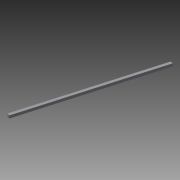
# Autodesk Inventor part: Stand
Saved by Autodesk Inventor 2017 (Build 210142000, 142)
## iProperties
Created: 2018-10-12
Part Number: Stand
Material: Wood (Birch)
Document SubType Name: Modeling
Designer: ari
Density: 0.55 g/cm^3
Appearance: Birch - Natural Polished
Author: ari
Autodesk Inventor part; units mm, degrees
ref_plane "XZ Plane" through (0, 0, 0) normal (0, 1, 0) x (-1, 0, 0)
ref_plane "XY Plane" through (0, 0, 0) normal (0, 0, 1) x (1, 0, 0)
sketch "Sketch1" plane through (0, 0, 0) normal (0, 0, 1) x (1, 0, 0)
  line L0 (-102.7252, -80.4997) -> (-34.2492, 156.7326)
  line L1 (-34.2492, 156.7326) -> (-39.0531, 158.1192)
  line L2 (-39.0531, 158.1192) -> (-107.529, -79.1131)
  line L3 (-107.529, -79.1131) -> (-102.7252, -80.4997)
  line L4 (-66.029, -80.4997) -> (-399.029, -80.4997) construction
  line L5 (-41.9395, 115.6973) -> (-41.9395, 350.8973) construction
  line L6 (-66.029, 141.7326) -> (-399.029, 141.7326) construction
  line L7 (-41.9395, 148.1192) -> (-41.9395, 158.1192) construction
  line L8 (-41.9395, 158.1192) -> (-39.0531, 158.1192) construction
  line L9 (-232.529, -80.4997) -> (-232.529, 141.7326) construction
  dimension "d0" = 5
  dimension "d1" = 15
  dimension "d2" = 10
  dimension "d3" = 125
  constraints: 14 end point, 3 point on line, 2 midpoint, 2 parallel, 2 perpendicular, 1 vertical
  measures "d0" distance of L2.end L0.start
  measures "d1" distance from line of L6 L0.end
  measures "d2" distance of L7.start L7.end
  measures "d3" distance from line of L9 L2.end
extrude "Extrusion1" add sketch "Sketch1" against normal blind 5
sketch "Sketch2" plane through (0, 0, 0) normal (0, 0, 1) x (1, 0, 0)
  line L0 (-102.7252, -80.4997) -> (-34.2492, 156.7326) projected
  line L1 (-34.2492, 156.7326) -> (-39.0531, 158.1192) projected
  line L2 (-39.0531, 158.1192) -> (-107.529, -79.1131) projected
  line L3 (-107.529, -79.1131) -> (-102.7252, -80.4997) projected
  point P0 (0, 0)
ref_plane "Work Plane1" through (-399.029, -65.6823, 68.7993) normal (0, -0.258819, -0.9659258) x (0, 0.9659258, -0.258819)
extrude "Extrusion2" add sketch "Sketch2" along normal up to surface surface through (-399.029, -65.6823, 68.7993) normal (0, -0.258819, -0.9659258)
ref_plane "Work Plane2" through (-34.2492, 156.7326, 9.2034) normal (1, 0, 0) x (0, 1, 0)
sketch "Sketch3" plane through (-34.2492, 156.7326, 9.2034) normal (1, 0, 0) x (0, 1, 0)
  line L0 (-8.6134, -9.2034) -> (-41.0353, -9.2034) construction
  line L1 (-41.0353, -9.2034) -> (-41.0353, -0.7034) construction
  line L2 (-41.0353, -0.7034) -> (-8.6134, -0.7034) construction
  line L3 (-8.6134, -0.7034) -> (-8.6134, -9.2034) construction
  line L4 (-8.6134, -0.7034) -> (-41.0353, -9.2034) construction
  line L5 (-41.4353, -0.3034) -> (-8.2134, -0.3034)
  line L6 (-8.2134, -0.3034) -> (-8.2134, -9.6034)
  line L7 (-8.2134, -9.6034) -> (-41.4353, -9.6034)
  line L8 (-41.4353, -9.6034) -> (-41.4353, -0.3034)
  line L9 (-41.4353, -0.3034) -> (-8.2134, -9.6034) construction
  line L10 (-8.2134, -0.3034) -> (-41.4353, -9.6034) construction
  point P0 (-156.7326, -9.2034)
  point P1 (-24.8243, -4.9534)
  dimension "d10" = 0.4
  dimension "d11" = 0.4
  constraints: 22 end point, 4 parallel, 3 midpoint, 2 horizontal, 2 perpendicular, 1 other
  measures "d10" distance between parallel lines of L7 L0
  measures "d11" distance between parallel lines of L6 L3
extrude "Extrusion3" cut sketch "Sketch3" against normal through all
sketch "Sketch4" plane through (-102.7252, -80.4997, 72.7696) normal (0.9607766, -0.2773235, 0) x (0, 0, -1)
  line L0 (63.8696, 203.7904) -> (63.8696, 238.3685) construction
  line L1 (73.1696, 238.3685) -> (73.1696, 203.7904) construction
  line L2 (77.7696, 246.9172) -> (77.7696, 0) construction
  line L3 (59.2696, 230.2273) -> (59.2696, 246.9172)
  line L4 (59.2696, 246.9172) -> (63.5662, 246.9172)
  line L5 (63.5662, 246.9172) -> (59.2696, 230.2273)
  line L6 (0, 0) -> (63.5662, 246.9172) construction
  line L7 (59.2696, 238.3685) -> (63.8696, 238.3685) construction
  line L8 (63.8696, 238.3685) -> (73.1696, 238.3685) construction
  line L9 (73.1696, 238.3685) -> (77.7696, 238.3685) construction
  point P0 (72.7696, 105.8303)
  constraints: 10 end point, 4 point on line, 2 collinear, 1 horizontal, 1 perpendicular, 1 vertical
extrude "Extrusion4" add sketch "Sketch4" against normal up to surface (5 mm away)
sketch "Sketch5" plane through (-38.8777, 140.6973, 13.5) normal (-0.0691396, -0.2395315, -0.9684236) x (-0.9607766, 0.2773235, 0)
  line L0 (5, 0) -> (5, 17.2341) projected
  line L1 (0, 17.2341) -> (5, 17.2341) projected
  line L2 (0, 0) -> (0, 17.2341) projected
  line L3 (0, 0) -> (5, 0) projected
  point P0 (-76.3715, -117.1033)
extrude "Extrusion5" add sketch "Sketch5" along normal up to next
body "Solid1"
